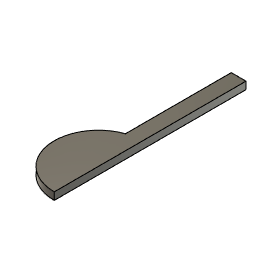
Démarreur v4 (Autodesk Fusion 360 design; units mm, degrees)
Autodesk Fusion 360 part; units mm, degrees
note: some values were not read from the file. Set by a fixed rule: which sketch regions a step uses.
sketch "Sketch1" plane through (0, 0, 0) normal (0, 1, 0) x (1, 0, 0)
  circle A0 centre (0, 0) radius 6
  line L0 (-2, 20) -> (2, 20)
  line L1 (2, 20) -> (2, 0)
  line L2 (2, 0) -> (-2, 0)
  line L3 (-2, 0) -> (-2, 20)
  line L4 (0, 20) -> (0, -6)
  dimension "d1" = 12
  dimension "d2" = 4
  dimension "d3" = 20
  constraint coincident A0.centre origin
  constraint horizontal L0
  constraint vertical L1
  constraint horizontal L2
  constraint vertical L3
  constraint midpoint A0.centre L2
  constraint midpoint L0 L4.start
  constraint coincident A0 L4.end
  constraint perpendicular L0 L4
  measures "d1" diameter of A0
  measures "d2" distance of L0.start L0.end
  measures "d3" distance of L0.start L2.end
extrude "Extrude1" add sketch "Sketch1" along normal blind 1 contours A0 L2 L3 L4 | A0 L0 L3 L4 | A0 L2 L3 L4
